Autodesk Inventor part; units mm, degrees
(part 5 of 5)
sketch "Эскиз48" plane through (1.5, -2, 18) normal (0, 0, 1) x (1, 0, 0)
  line L0 (0, 377) -> (-1.5, 377) projected
  line L1 (-17, 372.5031) -> (0, 323.3605)
  line L2 (0, 374) -> (0, 0) projected
  point P0 (-1.5, 2)
  dimension "d258" = 52
  dimension "d259" = 17
  constraints: 2 end point
  measures "d258" distance of L1.start L1.end
  measures "d259" distance from line of L1.start L2
sketch "Эскиз50" plane through (1.5, 0, 0) normal (1, 0, 0) x (0, 0, -1)
  arc A0 (291, 373) -> (289, 375) centre (289, 373) ccw projected
  line L0 (289, 375) -> (81, 375) projected
  arc A1 (81, 375) -> (79, 373) centre (81, 373) ccw projected
  line L1 (79, 373) -> (79, 320.5966) projected
  line L2 (79, 320.5966) -> (78, 320.5966) projected
  line L3 (78, 320.5966) -> (78, 372) projected
  arc A2 (78, 372) -> (75, 375) centre (75, 372) ccw projected
  line L4 (75, 375) -> (-15, 375) projected
  arc A3 (-15, 375) -> (-18, 372) centre (-15, 372) ccw projected
  line L5 (-18, 372) -> (-18, -2) projected
  arc A4 (-18, -2) -> (-15, -5) centre (-15, -2) ccw projected
  line L6 (-15, -5) -> (385, -5) projected
  arc A5 (385, -5) -> (388, -2) centre (385, -2) ccw projected
  line L7 (388, -2) -> (388, 372) projected
  arc A6 (388, 372) -> (385, 375) centre (385, 372) ccw projected
  line L8 (385, 375) -> (295, 375) projected
  arc A7 (295, 375) -> (292, 372) centre (295, 372) ccw projected
  line L9 (292, 372) -> (292, 320.5966) projected
  line L10 (292, 320.5966) -> (291, 320.5966) projected
  line L11 (291, 320.5966) -> (291, 373) projected
  line L12 (100.825, 134.3849) -> (78.75, 134.3849) projected
  line L13 (78.75, 134.3849) -> (78.75, 229.3849) projected
  line L14 (78.75, 229.3849) -> (100.825, 229.3849) projected
  line L15 (100.825, 229.3849) -> (100.825, 134.3849) projected
  circle A8 centre (56.2032, 142) radius 1.625 projected
  circle A9 centre (56.2032, 368) radius 1.625 projected
  circle A10 centre (73.2032, 228) radius 1.625 projected
  circle A11 centre (73.2032, 2.0002) radius 1.625 projected
  circle A12 centre (73.2032, 142) radius 1.625 projected
  circle A13 centre (73.2032, 368) radius 1.625 projected
  circle A14 centre (56.2032, 228) radius 1.625 projected
  circle A15 centre (56.2032, 2.0002) radius 1.625 projected
  circle A16 centre (313.7968, 142) radius 1.625 projected
  circle A17 centre (313.7968, 368) radius 1.625 projected
  circle A18 centre (296.7968, 228) radius 1.625 projected
  circle A19 centre (296.7968, 2.0002) radius 1.625 projected
  circle A20 centre (296.7968, 142) radius 1.625 projected
  circle A21 centre (296.7968, 368) radius 1.625 projected
  circle A22 centre (313.7968, 228) radius 1.625 projected
  circle A23 centre (313.7968, 2.0002) radius 1.625 projected
  arc A24 (330, 27.152) -> (328, 29.152) centre (328, 27.152) ccw projected
  line L16 (328, 29.152) -> (316, 29.152) projected
  arc A25 (314, 31.152) -> (316, 29.152) centre (316, 31.152) ccw projected
  line L17 (314, 31.152) -> (314, 107.152) projected
  arc A26 (316, 109.152) -> (314, 107.152) centre (316, 107.152) ccw projected
  line L18 (316, 109.152) -> (328, 109.152) projected
  arc A27 (328, 109.152) -> (330, 111.152) centre (328, 111.152) ccw projected
  line L19 (330, 111.152) -> (330, 160) projected
  arc A28 (333, 163) -> (330, 160) centre (333, 160) ccw projected
  line L20 (333, 163) -> (377, 163) projected
  arc A29 (380, 160) -> (377, 163) centre (377, 160) ccw projected
  line L21 (380, 160) -> (380, 3) projected
  arc A30 (377, 0) -> (380, 3) centre (377, 3) ccw projected
  line L22 (377, 0) -> (333, 0) projected
  arc A31 (330, 3) -> (333, 0) centre (333, 3) ccw projected
  line L23 (330, 3) -> (330, 27.152) projected
  arc A32 (328, 340.848) -> (330, 342.848) centre (328, 342.848) ccw projected
  line L24 (330, 342.848) -> (330, 367) projected
  arc A33 (333, 370) -> (330, 367) centre (333, 367) ccw projected
  line L25 (333, 370) -> (377, 370) projected
  arc A34 (380, 367) -> (377, 370) centre (377, 367) ccw projected
  line L26 (380, 367) -> (380, 262.848) projected
  arc A35 (378, 260.848) -> (380, 262.848) centre (378, 262.848) ccw projected
  line L27 (378, 260.848) -> (316, 260.848) projected
  arc A36 (314, 262.848) -> (316, 260.848) centre (316, 262.848) ccw projected
  line L28 (314, 262.848) -> (314, 338.848) projected
  arc A37 (316, 340.848) -> (314, 338.848) centre (316, 338.848) ccw projected
  line L29 (316, 340.848) -> (328, 340.848) projected
  arc A38 (40, 342.848) -> (42, 340.848) centre (42, 342.848) ccw projected
  line L30 (42, 340.848) -> (54, 340.848) projected
  arc A39 (56, 338.848) -> (54, 340.848) centre (54, 338.848) ccw projected
  line L31 (56, 338.848) -> (56, 262.848) projected
  arc A40 (54, 260.848) -> (56, 262.848) centre (54, 262.848) ccw projected
  line L32 (54, 260.848) -> (-8, 260.848) projected
  arc A41 (-10, 262.848) -> (-8, 260.848) centre (-8, 262.848) ccw projected
  line L33 (-10, 262.848) -> (-10, 367) projected
  arc A42 (-7, 370) -> (-10, 367) centre (-7, 367) ccw projected
  line L34 (-7, 370) -> (37, 370) projected
  arc A43 (40, 367) -> (37, 370) centre (37, 367) ccw projected
  line L35 (40, 367) -> (40, 342.848) projected
  arc A44 (42, 29.152) -> (40, 27.152) centre (42, 27.152) ccw projected
  line L36 (40, 27.152) -> (40, 3) projected
  arc A45 (37, 0) -> (40, 3) centre (37, 3) ccw projected
  line L37 (37, 0) -> (-7, 0) projected
  arc A46 (-10, 3) -> (-7, 0) centre (-7, 3) ccw projected
  line L38 (-10, 3) -> (-10, 160) projected
  arc A47 (-7, 163) -> (-10, 160) centre (-7, 160) ccw projected
  line L39 (-7, 163) -> (37, 163) projected
  arc A48 (40, 160) -> (37, 163) centre (37, 160) ccw projected
  line L40 (40, 160) -> (40, 111.152) projected
  arc A49 (40, 111.152) -> (42, 109.152) centre (42, 111.152) ccw projected
  line L41 (42, 109.152) -> (54, 109.152) projected
  arc A50 (56, 107.152) -> (54, 109.152) centre (54, 107.152) ccw projected
  line L42 (56, 107.152) -> (56, 31.152) projected
  arc A51 (54, 29.152) -> (56, 31.152) centre (54, 31.152) ccw projected
  line L43 (54, 29.152) -> (42, 29.152) projected
  circle A52 centre (103, 60) radius 2.1 projected
  circle A53 centre (135.25, 60) radius 2.1 projected
  circle A54 centre (173.9908, 56.343) radius 2.1 projected
  circle A55 centre (50.8872, 165.0002) radius 2.1 projected
  circle A56 centre (287, 56.343) radius 2.1 projected
  circle A57 centre (319.1128, 165.0002) radius 2.1 projected
  line L44 (165, 44) -> (165, 8) projected
  arc A58 (162, 5) -> (165, 8) centre (162, 8) ccw projected
  line L45 (162, 5) -> (96, 5) projected
  arc A59 (93, 8) -> (96, 5) centre (96, 8) ccw projected
  line L46 (93, 8) -> (93, 44) projected
  arc A60 (96, 47) -> (93, 44) centre (96, 44) ccw projected
  line L47 (96, 47) -> (162, 47) projected
  arc A61 (165, 44) -> (162, 47) centre (162, 44) ccw projected
  circle A62 centre (152.75, 251.9941) radius 2.1 projected
  circle A63 centre (217.25, 118.0059) radius 2.1 projected
  circle A64 centre (217.25, 57.0059) radius 2.1 projected
  circle A65 centre (217.25, 251.9941) radius 2.1 projected
  circle A66 centre (152.75, 312.9941) radius 2.1 projected
  circle A67 centre (152.75, 118.0059) radius 2.1 projected
  circle A68 centre (152.75, 57.0059) radius 2.1 projected
  circle A69 centre (217.25, 312.9941) radius 2.1 projected
  circle A70 centre (124.375, 193.0059) radius 2 projected
  circle A71 centre (124.375, 129.0059) radius 2 projected
  line L48 (358.5, 244.5001) -> (358.5, 185.5001) projected
  arc A72 (355.5, 182.5001) -> (358.5, 185.5001) centre (355.5, 185.5001) ccw projected
  line L49 (355.5, 182.5001) -> (335, 182.5001) projected
  arc A73 (332, 185.5001) -> (335, 182.5001) centre (335, 185.5001) ccw projected
  line L50 (332, 185.5001) -> (332, 244.5001) projected
  arc A74 (335, 247.5001) -> (332, 244.5001) centre (335, 244.5001) ccw projected
  line L51 (335, 247.5001) -> (355.5, 247.5001) projected
  arc A75 (358.5, 244.5001) -> (355.5, 247.5001) centre (355.5, 244.5001) ccw projected
  line L52 (14.5, 247.5001) -> (35, 247.5001) projected
  arc A76 (38, 244.5001) -> (35, 247.5001) centre (35, 244.5001) ccw projected
  line L53 (38, 244.5001) -> (38, 185.5001) projected
  arc A77 (35, 182.5001) -> (38, 185.5001) centre (35, 185.5001) ccw projected
  line L54 (35, 182.5001) -> (14.5, 182.5001) projected
  arc A78 (11.5, 185.5001) -> (14.5, 182.5001) centre (14.5, 185.5001) ccw projected
  line L55 (11.5, 185.5001) -> (11.5, 244.5001) projected
  arc A79 (14.5, 247.5001) -> (11.5, 244.5001) centre (14.5, 244.5001) ccw projected
  arc A80 (185, 193.309) -> (185, 192.7028) centre (183.175, 193.0059) ccw projected
  line L56 (185, 193.309) -> (185, 192.7028) projected
  circle A81 centre (183.175, 129.0059) radius 1.85 projected
  circle A82 centre (-9, 228) radius 1.625 projected
  circle A83 centre (379, 228) radius 1.625 projected
  circle A84 centre (-9.0468, 185.0848) radius 1.625 projected
  circle A85 centre (379.0468, 185.0848) radius 1.625 projected
  circle A86 centre (-13.6, 1.1) radius 1.625 projected
  circle A87 centre (383.6, 1.1) radius 1.625 projected
  circle A88 centre (-13.6, 369) radius 1.625 projected
  circle A89 centre (383.6, 368.9) radius 1.625 projected
  line L57 (46, 184.5001) -> (46, 245.5001)
  arc A90 (46, 244.5001) -> (35, 255.5001) centre (35, 244.5001) ccw
  line L58 (35, 255.5001) -> (14.5, 255.5001)
  arc A91 (14.5, 255.5001) -> (3.5, 244.5001) centre (14.5, 244.5001) ccw
  line L59 (3.5, 245.5001) -> (3.5, 184.5001)
  arc A92 (3.5, 185.5001) -> (14.5, 174.5001) centre (14.5, 185.5001) ccw
  line L60 (14.5, 174.5001) -> (35, 174.5001)
  arc A93 (35, 174.5001) -> (46, 185.5001) centre (35, 185.5001) ccw
  line L61 (44, 182.5001) -> (5.5, 182.5001)
  line L62 (38, 215.0001) -> (11.5, 215.0001)
  line L63 (44, 247.5001) -> (5.5, 247.5001)
  arc A94 (46, 245.5001) -> (44, 247.5001) centre (44, 245.5001) ccw
  arc A95 (5.5, 247.5001) -> (3.5, 245.5001) centre (5.5, 245.5001) ccw
  arc A96 (3.5, 184.5001) -> (5.5, 182.5001) centre (5.5, 184.5001) ccw
  arc A97 (44, 182.5001) -> (46, 184.5001) centre (44, 184.5001) ccw
  line L64 (185, 451.8698) -> (185, -81.8698) projected
  line L65 (324, 184.5001) -> (324, 245.5001)
  line L66 (366.5, 245.5001) -> (366.5, 184.5001)
  line L67 (326, 182.5001) -> (364.5, 182.5001)
  line L68 (326, 247.5001) -> (364.5, 247.5001)
  arc A98 (326, 247.5001) -> (324, 245.5001) centre (326, 245.5001) ccw
  arc A99 (366.5, 245.5001) -> (364.5, 247.5001) centre (364.5, 245.5001) ccw
  arc A100 (364.5, 182.5001) -> (366.5, 184.5001) centre (364.5, 184.5001) ccw
  arc A101 (324, 184.5001) -> (326, 182.5001) centre (326, 184.5001) ccw
  point P0 (0, 0)
  point P1 (45.583, 182.5001)
  point P2 (3.917, 182.5001)
  point P3 (45.583, 247.5001)
  point P4 (3.917, 247.5001)
  dimension "d274" = 8
  dimension "d275" = 2
  constraints: 26 point on circle, 22 end point, 14 symmetric about line, 12 centre point, 8 point on line, 8 tangent, 3 equal radius, 2 midpoint, 11 other
  measures "d274" distance between parallel lines of L53 L57
  measures "d275" radius of A94
extrude "Выдавливание41" cut sketch "Эскиз50" against normal blind 10 contours A75 L68 A99 L66 A100 L67 A72 L48 | L48 A72 L49 A73 L50 A74 L51 A75 | A74 L50 A73 L67 A101 L65 A98 L68 | L52 A76 L53 L62 L55 A79 | A79 L55 A78 L61 A96 A92 L59 A91 A95 L63 | L63 A94 A90 L57 A93 A97 L61 A77 L53 A76 | L62 L53 A77 L54 A78 L55 | A91 L59 A95 | A94 L57 A90 | A92 A96 L59 | L57 A97 A93
equation "\"d99\" = d97"
